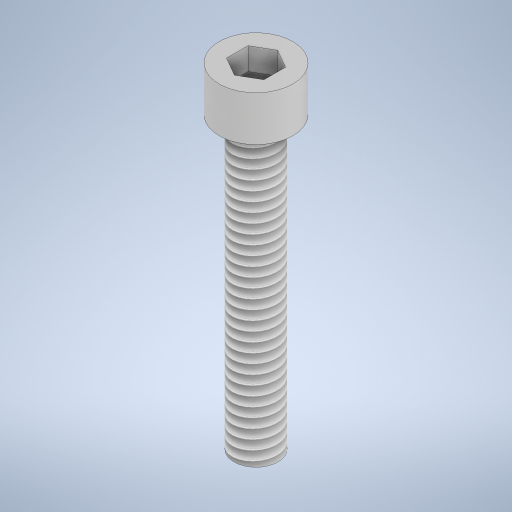
# Autodesk Inventor part: Threaded Rod Screw
Saved by Autodesk Inventor 2024 (Build 280153000, 153)
## iProperties
Created: 2023-06-07
Part Number: Threaded Rod Screw
Material: Generic
Document SubType Name: Modeling
Designer: 18179
Density: 1 g/cm^3
Appearance: Machined - Aluminum
Author: 18179
Autodesk Inventor part; units mm, degrees
ref_plane "YZ Plane" through (0, 0, 0) normal (1, 0, 0) x (0, 1, 0)
ref_plane "XZ Plane" through (0, 0, 0) normal (0, 1, 0) x (-1, 0, 0)
ref_plane "XY Plane" through (0, 0, 0) normal (0, 0, 1) x (1, 0, 0)
sketch "Sketch1" plane through (0, 0, 0) normal (0, 1, 0) x (-1, 0, 0)
  circle A0 centre (0, 0) radius 1.5
  dimension "d0" = 3
  constraints: 1 centre point, 1 coincident
  measures "d0" diameter of A0
extrude "Extrusion1" add sketch "Sketch1" along normal blind 19.685
sketch "Sketch2" plane through (0, 19.685, 0) normal (0, 1, 0) x (1, 0, 0)
  circle A0 centre (0, 0) radius 1.5 projected
  circle A1 centre (0, 0) radius 2.5
  dimension "d3" = 5
  constraints: 1 centre point, 1 coincident
  measures "d3" diameter of A1
extrude "Extrusion2" add sketch "Sketch2" along normal blind 3.048 contours A0 | A1
sketch "Sketch3" plane through (0, 22.733, 0) normal (0, 1, 0) x (1, 0, 0)
  circle A0 centre (0, 0) radius 2.5 projected
  line L0 (-1.27, 0.7332) -> (0, 1.4665)
  line L1 (0, 1.4665) -> (1.27, 0.7332)
  line L2 (1.27, 0.7332) -> (1.27, -0.7332)
  line L3 (1.27, -0.7332) -> (0, -1.4665)
  line L4 (0, -1.4665) -> (-1.27, -0.7332)
  line L5 (-1.27, -0.7332) -> (-1.27, 0.7332)
  dimension "d6" = 1.27
  constraints: 12 end point, 1 coincident, 13 other
  measures "d6" distance from line of point (0, 0) L5
extrude "Extrusion3" cut sketch "Sketch3" against normal blind 1.524 contours L0 L1 L2 L3 L4 L5
thread "Thread1" size "5-40 UNC" class "2A" standard "ANSI Unified Screw Threads" full length
body "Solid1"
